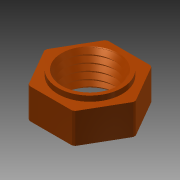
# Autodesk Inventor part: lock nut
Saved by Autodesk Inventor 2014 (Build 180170000, 170)
## iProperties
Created: 2013-07-23
Part Number: lock nut
Material: Generic
Document SubType Name: Modeling
Designer: employee
Density: 1 g/cm^3
Mass: 2.17902 g
Surface Area: 18.3194 cm^2
Volume: 2.17902 cm^3
Appearance: Smooth - Light Orange
Author: employee
Autodesk Inventor part; units mm, degrees
ref_plane "YZ Plane" through (0, 0, 0) normal (1, 0, 0) x (0, 1, 0)
ref_plane "XZ Plane" through (0, 0, 0) normal (0, 1, 0) x (-1, 0, 0)
ref_plane "XY Plane" through (0, 0, 0) normal (0, 0, 1) x (1, 0, 0)
sketch "Sketch1" plane through (0, 0, 0) normal (0, 0, 1) x (1, 0, 0)
  circle A0 centre (0, 0) radius 12.5
  dimension "d0" = 25
  constraints: 1 centre point, 1 coincident
  measures "d0" diameter of A0
extrude "Extrusion1" add sketch "Sketch1" along normal blind 10
sketch "Sketch2" plane through (0, 0, 10) normal (0, 0, 1) x (1, 0, 0)
  circle A0 centre (0, 0) radius 12.5 projected
  circle A1 centre (0, 0) radius 6.95
  dimension "d4" = 13.9
  constraints: 1 centre point, 1 coincident
  measures "d4" diameter of A1
extrude "Extrusion2" cut sketch "Sketch2" against normal through all contours A1
sketch "Sketch3" plane through (0, 0, 0) normal (0, 1, 0) x (-1, 0, 0)
  line L0 (12.5, 10) -> (12.5, 0) projected
  line L1 (12.5, 0) -> (6.95, 0) projected
  line L2 (6.95, 0) -> (6.95, 10) projected
  line L3 (6.95, 10) -> (12.5, 10) projected
  line L4 (-12.5, 0) -> (-12.5, 10) projected
  line L5 (-12.5, 10) -> (-6.95, 10) projected
  line L6 (-6.95, 10) -> (-6.95, 0) projected
  line L7 (-6.95, 0) -> (-12.5, 0) projected
  line L8 (-6.95, 10) -> (-6.95, 12)
  line L9 (0, 0) -> (0, 4.0318)
  line L10 (-6.95, 10) -> (-7.95, 11)
  line L11 (-7.95, 11) -> (-6.95, 12)
  dimension "d11" = 2
  constraints: 8 end point, 3 perpendicular, 1 parallel
  measures "d11" distance of L5.end L8.end
coil "Coil1" sketch "Sketch3" operation cut axis through (0, 0, 0) along (0, 0, -1) pitch 2.0001 turns 10 hand right contours L10 L11 L8
sketch "Sketch9" plane through (0, 0, 10) normal (0, 0, 1) x (1, 0, 0)
  circle A0 centre (0, 0) radius 12.5 projected
  circle A1 centre (0, 0) radius 9
  dimension "d47" = 18
  constraints: 1 centre point, 1 coincident
  measures "d47" diameter of A1
extrude "Extrusion8" cut sketch "Sketch9" against normal blind 1.5
sketch "Sketch10" plane through (0, 0, 10) normal (0, 0, 1) x (1, 0, 0)
  arc A0 (6.95, 0) -> (6.95, 0.0022) centre (0, 0) ccw projected
  circle A1 centre (0, 0) radius 7.95
  constraints: 1 centre point, 1 coincident
extrude "Extrusion9" cut sketch "Sketch10" against normal blind 5 draft -45
sketch "Sketch11" plane through (0, 0, 0) normal (0, 0, -1) x (-1, 0, 0)
  arc A0 (-6.95, 0.0131) -> (-6.95, 0.0109) centre (0, 0) ccw projected
  circle A1 centre (0, 0) radius 7.95
  constraints: 1 centre point, 1 coincident
extrude "Extrusion10" cut sketch "Sketch11" against normal blind 5 draft -45
sketch "Sketch12" plane through (0, 0, 0) normal (0, 0, -1) x (-1, 0, 0)
  circle A0 centre (0, 0) radius 7.95 projected
  circle A1 centre (0, 0) radius 12.5 projected
  line L0 (-12.7017, 0) -> (-6.3509, 11)
  line L1 (-6.3509, 11) -> (6.3509, 11)
  line L2 (6.3509, 11) -> (12.7017, 0)
  line L3 (12.7017, 0) -> (6.3509, -11)
  line L4 (6.3509, -11) -> (-6.3509, -11)
  line L5 (-6.3509, -11) -> (-12.7017, 0)
  point P0 (7.95, -0.0137)
  dimension "d55" = 22
  constraints: 12 end point, 1 coincident, 1 horizontal, 14 other
  measures "d55" distance between parallel lines of L4 L1
extrude "Extrusion11" cut sketch "Sketch12" along normal through all both and the other way through all contours A0 | A1 L3 L4 L5 L0 L1 L2 | A1 L2 L3 | A1 L1 L2 | L3 L4 A1 | A1 L0 L1 | L4 L5 A1 | A1 L5 L0 keep common part
body "Solid1"
